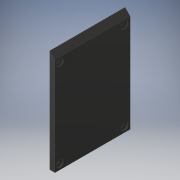
# Autodesk Inventor part: Deckel_2_Frame
Saved by Autodesk Inventor 2019 (Build 230136000, 136)
## iProperties
Created: 2021-11-06
Part Number: Deckel_2_Frame
Material: PC/ABS-Kunststoff
Document SubType Name: Modeling
Designer: Bergi
Density: 0.357273 g/cm^3
Appearance: Glatt - Schwarz
Mass: 12.5506 g
Surface Area: 163.174 cm^2
Volume: 35.1288 cm^3
Author: Bergi
Autodesk Inventor part; units mm, degrees
ref_plane "YZ Plane" through (0, 0, 0) normal (1, 0, 0) x (0, 1, 0)
ref_plane "XZ Plane" through (0, 0, 0) normal (0, 1, 0) x (-1, 0, 0)
ref_plane "XY Plane" through (0, 0, 0) normal (0, 0, 1) x (1, 0, 0)
sketch "Skizze1" plane through (0, 0, 0) normal (1, 0, 0) x (0, 1, 0)
  line L0 (-50, 36.5) -> (50, 36.5)
  line L1 (50, 36.5) -> (50, -36.5)
  line L2 (50, -36.5) -> (-50, -36.5)
  line L3 (-50, -36.5) -> (-50, 36.5)
  line L4 (-50, 36.5) -> (50, -36.5) construction
  line L5 (50, 36.5) -> (-50, -36.5) construction
  point P0 (0, 0)
  dimension "d0" = 73
  dimension "d1" = 100
  constraints: 12 end point, 2 midpoint, 2 parallel, 1 horizontal, 1 perpendicular
  measures "d0" distance of L0.end L1.end
  measures "d1" distance of L0.start L0.end
extrude "Extrusion1" add sketch "Skizze1" along normal blind 5
chamfer "Fase1" distance 5 angle 45 1 edges at (5, 50, 0)
sketch "Skizze2" plane through (5, 0, 0) normal (1, 0, 0) x (0, 0, -1)
  line L0 (-36.5, 45) -> (-36.5, -50) projected
  line L1 (-36.5, 45) -> (36.5, 45) projected
  line L2 (-36.5, -50) -> (36.5, -50) projected
  line L3 (0, -70) -> (0, 70) construction
  point P0 (0, 0)
  point P1 (-31.5, -45)
  point P2 (-31.5, 40)
  point P3 (31.5, -45)
  point P4 (31.5, 40)
  dimension "d7" = 5
  dimension "d8" = 5
  dimension "d9" = 5
  dimension "d10" = 5
  constraints: 2 symmetric about line
  measures "d7" distance from line of L0 point (-31.5, 40)
  measures "d8" distance from line of L1 point (-31.5, 40)
  measures "d9" distance from line of L0 point (-31.5, -45)
  measures "d10" distance from line of L2 point (-31.5, -45)
hole "Bohrung1" at (5, -45, 31.5) at (5, 40, 31.5) at (5, 40, -31.5) at (5, -45, -31.5) direction (-1, 0, 0) diameter 4 end through all counterbore diameter 7 counterbore depth 2
